Autodesk Inventor part; units mm, degrees
(part 2 of 2)
  spline S158 degree 2 poles (35.0153, -80.3585) (36.3738, -80.3585) (37.8198, -81.6553) (37.8198, -82.8542) knots 0 0 0 1 2 2 2
  spline S159 degree 2 poles (37.8198, -82.8542) (37.8198, -84.0275) (36.4715, -85.4272) (35.2571, -85.4272) knots 0 0 0 1 2 2 2
  spline S160 degree 2 poles (35.2571, -85.4272) (34.161, -85.4272) (33.0495, -84.2385) (33.0495, -83.1373) knots 0 0 0 1 2 2 2
  line L114 (33.0495, -83.1373) -> (33.0495, -82.5969)
  line L115 (33.0495, -82.5969) -> (36.3275, -82.5969)
  spline S161 degree 2 poles (36.3275, -82.5969) (36.3069, -82.2625) (36.065, -81.8199) (35.8695, -81.6861) knots 0 0 0 1 2 2 2
  spline S162 degree 2 poles (35.8695, -81.6861) (35.6791, -81.5523) (35.1645, -81.4391) (34.8609, -81.4391) knots 0 0 0 1 2 2 2
  spline S163 degree 2 poles (34.8609, -81.4391) (34.6036, -81.4391) (34.0993, -81.5523) (33.8883, -81.6501) knots 0 0 0 1 2 2 2
  spline S164 degree 2 poles (33.8883, -81.6501) (33.7031, -81.7273) (33.3943, -81.9177) (33.2965, -81.9897) knots 0 0 0 1 2 2 2
  line L116 (33.2965, -81.9897) -> (33.137, -81.9897)
  line L117 (33.137, -81.9897) -> (33.137, -80.7547)
  spline S165 degree 2 poles (33.137, -80.7547) (33.3223, -80.6827) (33.6207, -80.5592) (33.8883, -80.4974) knots 0 0 0 1 2 2 2
  spline S166 degree 2 poles (33.8883, -80.4974) (34.1302, -80.4305) (34.6448, -80.3585) (35.0153, -80.3585) knots 0 0 0 1 2 2 2
  spline S167 degree 2 poles (34.5213, -83.4975) (34.5315, -83.9709) (34.9484, -84.47) (35.3755, -84.47) knots 0 0 0 1 2 2 2
  spline S168 degree 2 poles (35.3755, -84.47) (35.8129, -84.47) (36.3069, -83.9452) (36.3326, -83.4975) knots 0 0 0 1 2 2 2
  line L118 (36.3326, -83.4975) -> (34.5213, -83.4975)
  line L119 (58.9821, -76.3562) -> (61.164, -70.0062)
  line L120 (61.164, -70.0062) -> (62.8261, -70.0062)
  line L121 (62.8261, -70.0062) -> (65.0079, -76.3562)
  line L122 (65.0079, -76.3562) -> (63.3561, -76.3562)
  line L123 (63.3561, -76.3562) -> (61.9719, -72.0491)
  line L124 (61.9719, -72.0491) -> (60.5928, -76.3562)
  line L125 (60.5928, -76.3562) -> (58.9821, -76.3562)
  spline S169 degree 2 poles (53.687, -73.1812) (53.687, -72.3578) (53.9495, -71.1228) (54.2428, -70.706) knots 0 0 0 1 2 2 2
  spline S170 degree 2 poles (54.2428, -70.706) (54.531, -70.2943) (55.4624, -69.8724) (56.1313, -69.8724) knots 0 0 0 1 2 2 2
  spline S171 degree 2 poles (56.1313, -69.8724) (56.8054, -69.8724) (57.7317, -70.2943) (58.025, -70.7163) knots 0 0 0 1 2 2 2
  spline S172 degree 2 poles (58.025, -70.7163) (58.3183, -71.1331) (58.5808, -72.3578) (58.5808, -73.1812) knots 0 0 0 1 2 2 2
  spline S173 degree 2 poles (58.5808, -73.1812) (58.5808, -74.0251) (58.3183, -75.2189) (58.0199, -75.6512) knots 0 0 0 1 2 2 2
  spline S174 degree 2 poles (58.0199, -75.6512) (57.7214, -76.0731) (56.7797, -76.4848) (56.1313, -76.4848) knots 0 0 0 1 2 2 2
  spline S175 degree 2 poles (56.1313, -76.4848) (55.4469, -76.4848) (54.531, -76.0525) (54.2376, -75.6254) knots 0 0 0 1 2 2 2
  spline S176 degree 2 poles (54.2376, -75.6254) (53.9495, -75.2086) (53.687, -73.9788) (53.687, -73.1812) knots 0 0 0 1 2 2 2
  spline S177 degree 2 poles (55.2874, -73.1812) (55.2874, -74.3596) (55.6733, -75.3115) (56.1313, -75.3115) knots 0 0 0 1 2 2 2
  spline S178 degree 2 poles (56.1313, -75.3115) (56.5893, -75.3115) (56.9804, -74.3596) (56.9804, -73.176) knots 0 0 0 1 2 2 2
  spline S179 degree 2 poles (56.9804, -73.176) (56.9804, -72.013) (56.5893, -71.0456) (56.1313, -71.0456) knots 0 0 0 1 2 2 2
  spline S180 degree 2 poles (56.1313, -71.0456) (55.6785, -71.0456) (55.2874, -72.013) (55.2874, -73.1812) knots 0 0 0 1 2 2 2
  line L126 (48.042, -70.0062) -> (52.7093, -70.0062)
  line L127 (52.7093, -70.0062) -> (52.7093, -71.0405)
  spline S181 degree 2 poles (52.7093, -71.0405) (52.1175, -71.5139) (51.1707, -72.3475) (50.8156, -72.7232) knots 0 0 0 1 2 2 2
  spline S182 degree 2 poles (50.8156, -72.7232) (50.3474, -73.212) (49.9306, -73.9582) (49.9306, -74.3493) knots 0 0 0 1 2 2 2
  spline S183 degree 2 poles (49.9306, -74.3493) (49.9306, -74.7918) (50.4606, -75.2652) (50.934, -75.2652) knots 0 0 0 1 2 2 2
  spline S184 degree 2 poles (50.934, -75.2652) (51.1759, -75.2652) (51.6081, -75.1469) (51.8294, -75.0542) knots 0 0 0 1 2 2 2
  spline S185 degree 2 poles (51.8294, -75.0542) (52.0455, -74.9565) (52.3543, -74.7506) (52.4314, -74.6992) knots 0 0 0 1 2 2 2
  line L128 (52.4314, -74.6992) -> (52.5549, -74.6992)
  line L129 (52.5549, -74.6992) -> (52.5549, -76.0834)
  spline S186 degree 2 poles (52.5549, -76.0834) (52.2874, -76.2121) (51.145, -76.4797) (50.615, -76.4797) knots 0 0 0 1 2 2 2
  spline S187 degree 2 poles (50.615, -76.4797) (49.4829, -76.4797) (48.3199, -75.4711) (48.3199, -74.5602) knots 0 0 0 1 2 2 2
  spline S188 degree 2 poles (48.3199, -74.5602) (48.3199, -73.9993) (48.8499, -72.9187) (49.4623, -72.3012) knots 0 0 0 1 2 2 2
  spline S189 degree 2 poles (49.4623, -72.3012) (49.8482, -71.9204) (50.5738, -71.3286) (50.7333, -71.2051) knots 0 0 0 1 2 2 2
  line L130 (50.7333, -71.2051) -> (48.042, -71.2051)
  line L131 (48.042, -71.2051) -> (48.042, -70.0062)
  point P0 (56.4324, -6.35)
  constraints: 2 end point, 2 midpoint, 1 horizontal
extrude "Name and Version Number" cut sketch "Sketch15" against normal blind 3.175
equation "\"d14\" = gapBetweenParts"
equation "\"d16\" = gapBetweenParts"
equation "\"d18\" = gapBetweenParts"
equation "\"d20\" = gapBetweenParts"
equation "\"d21\" = gapBetweenParts"
equation "\"gapBetweenParts\" = 7.9375"
body "Solid3"
